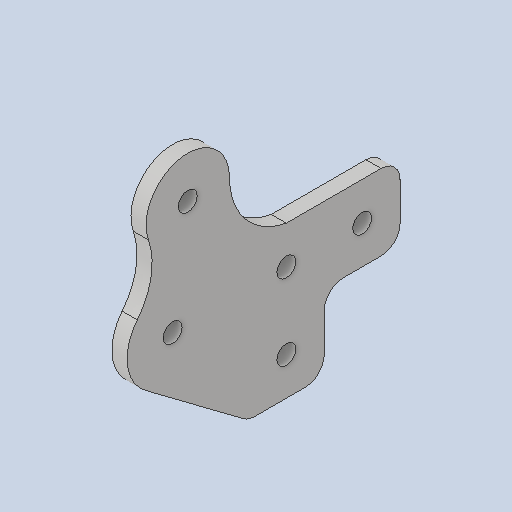
# Autodesk Inventor part: KettenBlech_Oben
Saved by Autodesk Inventor 2022 (Build 260153000, 153)
## iProperties
Created: 2020-01-07
Part Number: KettenBlech_Oben
Material: Generisch
Document SubType Name: Modeling
Designer: kaebi
Density: 1 g/cm^3
Appearance: Vorgabe
Description: Aufnahme Umlenkung (Bestand)
Stock Number: -
Author: kaebi
Autodesk Inventor part; units mm, degrees
ref_plane "YZ Plane" through (0, 0, 0) normal (1, 0, 0) x (0, 1, 0)
ref_plane "XZ Plane" through (0, 0, 0) normal (0, 1, 0) x (-1, 0, 0)
ref_plane "XY Plane" through (0, 0, 0) normal (0, 0, 1) x (1, 0, 0)
sketch "Skizze1" plane through (0, 0, 0) normal (1, 0, 0) x (0, 1, 0)
  line L0 (-30, 10) -> (-30, -10)
  arc A0 (28, 15) -> (24.3693, 36.3836) centre (28, 26) ccw
  line L1 (-9.6, 37.2) -> (-30, 10)
  line L2 (10, -3) -> (10, 0)
  arc A1 (28, 15) -> (10, 0) centre (28, -3.3) ccw
  line L3 (-10, -30) -> (10, -30)
  line L4 (10, -30) -> (10, 0)
  line L5 (-10, -10) -> (-30, -10)
  line L6 (-10, -10) -> (-10, -30)
  arc A2 (7.5634, 39.3164) -> (24.3693, 36.3836) centre (18.5933, 52.9028) ccw
  arc A3 (7.5634, 39.3164) -> (-9.6, 37.2) centre (0, 30) ccw
  point P0 (0, 0)
  point P1 (-30, 0)
  dimension "d16" = 22
  dimension "d22" = 10
  dimension "d23" = 18
  dimension "d26" = 30
  dimension "d31" = 20
  dimension "d34" = 26
  dimension "d35" = 10
  dimension "d36" = 20
  dimension "d37" = 18
  dimension "d38" = 18
  dimension "d39" = 0
  dimension "d40" = 30
  dimension "d43" = 35
  dimension "d44" = 12
  dimension "d46" = 0
  constraints: 14 end point, 8 point on circle, 4 centre point, 3 tangent, 3 vertical, 1 horizontal, 1 horizontal alignment, 1 midpoint, 1 parallel, 1 point on line
  measures "d16" diameter of A0
  measures "d22" distance from line of L2 point (0, 0)
  measures "d23" distance from line of A0.centre L2
  measures "d26" distance from line of L0 point (0, 0)
  measures "d31" distance between parallel lines of L3 L5
  measures "d34" vertical distance of point (0, 0) A0.centre
  measures "d35" distance from line of L5 point (0, 0)
  measures "d36" distance between parallel lines of L6 L4
  measures "d37" distance from line of L4 A0.start
  measures "d38" distance from line of L4 A1.centre
  measures "d39" vertical distance of point (0, 0) L2.end
  measures "d40" distance of A3.centre point (0, 0)
  measures "d43" diameter of A2
  measures "d44" radius of A3
  measures "d46" horizontal distance of A3.centre point (0, 0)
extrude "Extrusion1" add sketch "Skizze1" along normal mid plane 4
sketch "Skizze2" plane through (2, 0, 0) normal (1, 0, 0) x (0, 0, -1)
  circle A0 centre (-26, 28) radius 2.5
  circle A1 centre (0, 0) radius 2.5
  circle A2 centre (20, 0) radius 2.5
  circle A3 centre (0, -20) radius 2.5
  line L0 (-10, -30) -> (10, -30) projected
  line L1 (30, -10) -> (30, 10) projected
  arc A4 (-15, 28) -> (-36.3836, 24.3693) centre (-26, 28) ccw projected
  circle A5 centre (-30, 0) radius 2.5
  arc A6 (-39.3164, 7.5634) -> (-37.2, -9.6) centre (-30, 0) ccw projected
  point P0 (10, -27)
  point P1 (-36.9988, 28.1611)
  point P2 (-44.9983, -10.001)
  dimension "d8" = 5
  dimension "d9" = 5
  dimension "d10" = 5
  dimension "d11" = 10
  dimension "d32" = 10
  dimension "d45" = 5
  constraints: 5 centre point, 2 coincident, 1 concentric, 1 equal radius, 1 horizontal alignment, 1 vertical alignment, 2 other
  measures "d8" diameter of A0
  measures "d9" diameter of A1
  measures "d10" diameter of A3
  measures "d11" distance from line of A3.centre L0
  measures "d32" distance from line of A2.centre L1
  measures "d45" diameter of A5
extrude "Extrusion2" cut sketch "Skizze2" along normal through all both and the other way through all
fillet "Fillet1" radius 5 5 edges at (0, -30, -10) (0, -10, -10) (0, -10, -30) (0, 10, -30) (0, -30, 10)
